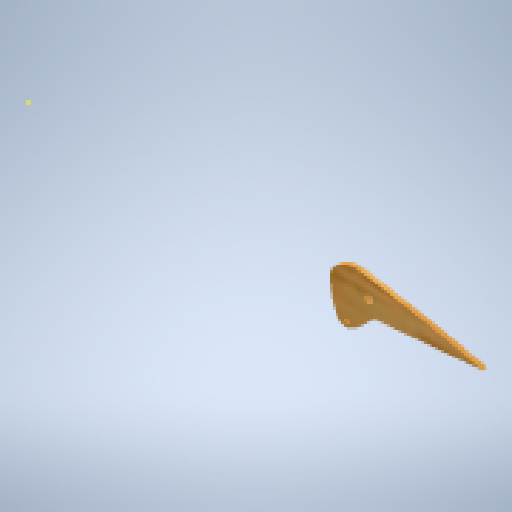
# Autodesk Inventor part: AIL middle connecting rib extension assembly
Saved by Autodesk Inventor 2025.2 (Build 292293000, 293)
## iProperties
Created: 2024-11-18
Part Number: AIL middle connecting rib extension assembly
Material: Plywood, Finish
Document SubType Name: Modeling
Designer: thoma
Density: 0.552 g/cm^3
Appearance: Plywood - New
Author: thoma
Autodesk Inventor part; units mm, degrees
ref_plane "YZ Plane" through (0, 0, 0) normal (1, 0, 0) x (0, 1, 0)
ref_plane "XZ Plane" through (0, 0, 0) normal (0, 1, 0) x (-1, 0, 0)
ref_plane "XY Plane" through (0, 0, 0) normal (0, 0, 1) x (1, 0, 0)
sketch "Sketch1" plane through (0, 0, 0) normal (0, 0, 1) x (1, 0, 0)
  spline S0 degree 4 poles (227.9538, -6.6666) (233.9795, -6.1502) (242.1312, -5.4418) (252.1108, -4.5554) (263.3906, -3.5266) (270.7075, -2.8494) (277.2598, -2.2283) (283.0709, -1.6797) (287.955, -1.1879) (292.1861, -0.8066) (295.1251, -0.4496) (297.859, -0.2789) (298.9117, -0.0313) (300.6417, -0.0427) (298.9253, 0.1752) (297.9143, 0.5599) (295.2242, 1.0851) (292.3531, 1.8178) (288.198, 2.7284) (283.4022, 3.8159) (277.6828, 5.0504) (271.2241, 6.4164) (263.9961, 7.8887) (256.0707, 9.4454) (247.4873, 11.0611) (237.0929, 12.9289) (228.6426, 14.3598) (222.3187, 15.3801) (218.5257, 15.9738) knots 0 0 0 0 0 0.123617 0.170541 0.215522 0.258317 0.298656 0.336232 0.370677 0.401524 0.428109 0.449222 0.465805 0.481001 0.497585 0.518702 0.545296 0.576159 0.61063 0.648244 0.688637 0.731505 0.776579 0.823621 0.872406 0.922727 1 1 1 1 1
  line L0 (200, 103) -> (200, -97) construction
  line L1 (300, -103) -> (300, 103) construction
  line L2 (200, 3.7134) -> (300, 0) construction
  circle A0 centre (225, 2.7851) radius 2.5
  line L3 (230.0222, 14.1744) -> (207.0292, 17.7732) construction
  arc A1 (227.7164, 14.4946) -> (209.3226, 17.3735) centre (52.1769, -1046.8526) ccw construction
  spline S1 degree 4 poles (200, 3.7134) (200.1429, 9.1319) (206.2023, 15.2323) (212.1452, 16.2028) (218.5257, 15.9738) knots 0 0 0 0 0 1 1 1 1 1
  line L4 (212.7843, 16.1798) -> (224.2671, 15.7678) construction
  arc A2 (223.0893, 15.5881) -> (213.9461, 15.9162) centre (216.8298, -31.2827) ccw construction
  line L5 (199.8716, -1.156) -> (200.1284, 8.5828) construction
  arc A3 (200.9996, 7.0523) -> (200.8223, 0.3265) centre (206.6628, 3.5377) ccw construction
  spline S2 degree 2 poles (227.9538, -6.6666) (202.7705, -38.1054) (200, 3.7134) knots 0 0 0 1 1 1
  circle A4 centre (211, -16.584) radius 1.5
  line L6 (197, -35.9531) -> (225, 2.7851) construction
  point P0 (299.5428, 0.1089)
  point P1 (298.1739, 0.4338)
  point P2 (295.9008, 0.9681)
  point P3 (292.7367, 1.7025)
  point P4 (288.6996, 2.6229)
  point P5 (283.8129, 3.7134)
  point P6 (278.1048, 4.9545)
  point P7 (271.6086, 6.3255)
  point P8 (264.3621, 7.8039)
  point P9 (256.4085, 9.3663)
  point P10 (247.7946, 10.9887)
  point P11 (238.572, 12.6468)
  point P12 (228.7959, 14.3166)
  point P13 (207.8235, 17.5944)
  point P14 (247.0398, -5.0019)
  point P15 (255.7236, -4.2234)
  point P16 (263.7597, -3.4905)
  point P17 (271.0965, -2.8098)
  point P18 (277.6872, -2.1882)
  point P19 (283.4889, -1.6323)
  point P20 (288.4641, -1.1487)
  point P21 (292.5804, -0.7434)
  point P22 (295.8102, -0.4221)
  point P23 (298.1328, -0.1887)
  point P24 (299.5323, -0.0474)
  point P25 (208.6203, -19.8763)
  dimension "d17" = 100
  dimension "d22" = 5
  dimension "d23" = 75
  dimension "d36" = 3
  constraints: 14 end point, 8 midpoint, 5 centre point, 3 point on circle, 3 point on line, 2 vertical, 41 other
  measures "d17" distance between parallel lines of L1 L0
  measures "d22" diameter of A0
  measures "d23" distance from line of L1 L6.end
  measures "d36" diameter of A4
sketch "Sketch3" plane through (0, 0, 0) normal (0, 0, 1) x (1, 0, 0)
  point P0 (0, 0)
sketch "Sketch4" plane through (0, 0, 0) normal (0, 0, 1) x (1, 0, 0)
  point P0 (0, 0)
sketch "Sketch5" plane through (0, 0, 0) normal (0, 0, 1) x (1, 0, 0)
  point P0 (0, 0)
sketch "Sketch6" plane through (0, 0, 0) normal (0, 0, 1) x (1, 0, 0)
  point P0 (0, 0)
sketch "Sketch7" plane through (0, 0, 0) normal (0, 0, 1) x (1, 0, 0)
  point P0 (0, 0)
sketch "Sketch8" plane through (0, 0, 0) normal (0, 0, 1) x (1, 0, 0)
  point P0 (0, 0)
extrude "Extrusion2" add sketch "Sketch1" along normal blind 3
body "Solid2"
